Autodesk Inventor part; units mm, degrees
(part 5 of 8)
  spline S575 degree 2 poles (-11.5089, 13.7039) (-11.2834, 13.8253) (-11.2834, 14.1341) knots 0 0 0 1 1 1
  line L2030 (-11.5089, 13.7039) -> (-11.2834, 13.8253) construction
  line L2031 (-11.2834, 13.8253) -> (-11.2834, 14.1341) construction
  spline S576 degree 2 poles (-11.2834, 14.1341) (-11.2834, 14.4706) (-11.5297, 14.651) knots 0 0 0 1 1 1
  line L2032 (-11.2834, 14.1341) -> (-11.2834, 14.4706) construction
  line L2033 (-11.2834, 14.4706) -> (-11.5297, 14.651) construction
  line L2034 (-11.5297, 14.651) -> (-13.0701, 15.7924)
  spline S577 degree 2 poles (-13.0701, 15.7924) (-13.3546, 16.0006) (-13.3546, 16.3787) knots 0 0 0 1 1 1
  line L2035 (-13.0701, 15.7924) -> (-13.3546, 16.0006) construction
  line L2036 (-13.3546, 16.0006) -> (-13.3546, 16.3787) construction
  spline S578 degree 2 poles (-13.3546, 16.3787) (-13.3546, 16.8748) (-12.8932, 17.1177) knots 0 0 0 1 1 1
  line L2037 (-13.3546, 16.3787) -> (-13.3546, 16.8748) construction
  line L2038 (-13.3546, 16.8748) -> (-12.8932, 17.1177) construction
  spline S579 degree 2 poles (-12.8932, 17.1177) (-12.5601, 17.2877) (-12.1403, 17.2877) knots 0 0 0 1 1 1
  line L2039 (-12.8932, 17.1177) -> (-12.5601, 17.2877) construction
  line L2040 (-12.5601, 17.2877) -> (-12.1403, 17.2877) construction
  spline S580 degree 2 poles (-12.1403, 17.2877) (-11.5159, 17.2877) (-11.0232, 16.9373) knots 0 0 0 1 1 1
  line L2041 (-12.1403, 17.2877) -> (-11.5159, 17.2877) construction
  line L2042 (-11.5159, 17.2877) -> (-11.0232, 16.9373) construction
  spline S581 degree 2 poles (-11.0232, 16.9373) (-10.9295, 16.8714) (-10.9295, 16.7708) knots 0 0 0 1 1 1
  line L2043 (-11.0232, 16.9373) -> (-10.9295, 16.8714) construction
  line L2044 (-10.9295, 16.8714) -> (-10.9295, 16.7708) construction
  spline S582 degree 2 poles (-2.041, 23.007) (-1.9282, 23.007) (-1.7632, 23.172) (-1.7632, 23.2848) knots 0 0 0 1 2 2 2
  line L2045 (-2.041, 23.007) -> (-1.9282, 23.007) construction
  line L2046 (-1.9282, 23.007) -> (-1.7632, 23.172) construction
  line L2047 (-1.7632, 23.172) -> (-1.7632, 23.2848) construction
  line L2048 (-1.7632, 23.2848) -> (-1.7632, 24.2529)
  spline S583 degree 2 poles (-1.7632, 24.2529) (-1.7632, 24.3656) (-1.9282, 24.5306) (-2.041, 24.5306) knots 0 0 0 1 2 2 2
  line L2049 (-1.7632, 24.2529) -> (-1.7632, 24.3656) construction
  line L2050 (-1.7632, 24.3656) -> (-1.9282, 24.5306) construction
  line L2051 (-1.9282, 24.5306) -> (-2.041, 24.5306) construction
  spline S584 degree 2 poles (-2.6405, 21.8326) (-2.6405, 21.6236) (-2.8496, 21.6236) knots 0 0 0 1 1 1
  line L2052 (-2.6405, 21.8326) -> (-2.6405, 21.6236) construction
  line L2053 (-2.6405, 21.6236) -> (-2.8496, 21.6236) construction
  spline S585 degree 2 poles (-2.8496, 21.6236) (-3.0586, 21.6236) (-3.0586, 21.8326) knots 0 0 0 1 1 1
  line L2054 (-2.8496, 21.6236) -> (-3.0586, 21.6236) construction
  line L2055 (-3.0586, 21.6236) -> (-3.0586, 21.8326) construction
  line L2056 (-3.0586, 21.8326) -> (-3.0586, 24.7369)
  spline S586 degree 2 poles (-3.0586, 24.7369) (-3.0586, 24.9459) (-2.8496, 24.9459) knots 0 0 0 1 1 1
  line L2057 (-3.0586, 24.7369) -> (-3.0586, 24.9459) construction
  line L2058 (-3.0586, 24.9459) -> (-2.8496, 24.9459) construction
  line L2059 (-2.8496, 24.9459) -> (-2.041, 24.9459)
  spline S587 degree 2 poles (-2.041, 24.9459) (-1.7522, 24.9459) (-1.3452, 24.5389) (-1.3452, 24.2529) knots 0 0 0 1 2 2 2
  line L2060 (-2.041, 24.9459) -> (-1.7522, 24.9459) construction
  line L2061 (-1.7522, 24.9459) -> (-1.3452, 24.5389) construction
  line L2062 (-1.3452, 24.5389) -> (-1.3452, 24.2529) construction
  line L2063 (-1.3452, 24.2529) -> (-1.3452, 23.2848)
  spline S588 degree 2 poles (-1.3452, 23.2848) (-1.3452, 22.9987) (-1.7522, 22.5917) (-2.041, 22.5917) knots 0 0 0 1 2 2 2
  line L2064 (-1.3452, 23.2848) -> (-1.3452, 22.9987) construction
  line L2065 (-1.3452, 22.9987) -> (-1.7522, 22.5917) construction
  line L2066 (-1.7522, 22.5917) -> (-2.041, 22.5917) construction
  spline S589 degree 2 poles (0.2225, 23.007) (0.3353, 23.007) (0.5003, 23.172) (0.5003, 23.2848) knots 0 0 0 1 2 2 2
  line L2067 (0.2225, 23.007) -> (0.3353, 23.007) construction
  line L2068 (0.3353, 23.007) -> (0.5003, 23.172) construction
  line L2069 (0.5003, 23.172) -> (0.5003, 23.2848) construction
  spline S590 degree 2 poles (-0.102, 24.5306) (-0.2148, 24.5306) (-0.3771, 24.3684) (-0.3771, 24.2529) knots 0 0 0 1 2 2 2
  line L2070 (-0.102, 24.5306) -> (-0.2148, 24.5306) construction
  line L2071 (-0.2148, 24.5306) -> (-0.3771, 24.3684) construction
  line L2072 (-0.3771, 24.3684) -> (-0.3771, 24.2529) construction
  line L2073 (-0.3771, 24.2529) -> (-0.3771, 23.2848)
  spline S591 degree 2 poles (-0.3771, 23.2848) (-0.3771, 23.1693) (-0.2148, 23.007) (-0.102, 23.007) knots 0 0 0 1 2 2 2
  line L2074 (-0.3771, 23.2848) -> (-0.3771, 23.1693) construction
  line L2075 (-0.3771, 23.1693) -> (-0.2148, 23.007) construction
  line L2076 (-0.2148, 23.007) -> (-0.102, 23.007) construction
  line L2077 (-0.102, 23.007) -> (0.2225, 23.007)
  line L2078 (0.2225, 22.5917) -> (-0.102, 22.5917)
  spline S592 degree 2 poles (-0.102, 22.5917) (-0.3881, 22.5917) (-0.7951, 22.996) (-0.7951, 23.2848) knots 0 0 0 1 2 2 2
  line L2079 (-0.102, 22.5917) -> (-0.3881, 22.5917) construction
  line L2080 (-0.3881, 22.5917) -> (-0.7951, 22.996) construction
  line L2081 (-0.7951, 22.996) -> (-0.7951, 23.2848) construction
  line L2082 (-0.7951, 23.2848) -> (-0.7951, 24.2529)
  spline S593 degree 2 poles (-0.7951, 24.2529) (-0.7951, 24.5417) (-0.3853, 24.9459) (-0.102, 24.9459) knots 0 0 0 1 2 2 2
  line L2083 (-0.7951, 24.2529) -> (-0.7951, 24.5417) construction
  line L2084 (-0.7951, 24.5417) -> (-0.3853, 24.9459) construction
  line L2085 (-0.3853, 24.9459) -> (-0.102, 24.9459) construction
  line L2086 (-0.102, 24.9459) -> (0.7065, 24.9459)
  spline S594 degree 2 poles (0.7065, 24.9459) (0.9183, 24.9459) (0.9183, 24.7369) knots 0 0 0 1 1 1
  line L2087 (0.7065, 24.9459) -> (0.9183, 24.9459) construction
  line L2088 (0.9183, 24.9459) -> (0.9183, 24.7369) construction
  line L2089 (0.9183, 24.7369) -> (0.9183, 23.2875)
  spline S595 degree 2 poles (0.9183, 23.2875) (0.9183, 23.0758) (1.0751, 22.996) knots 0 0 0 1 1 1
  line L2090 (0.9183, 23.2875) -> (0.9183, 23.0758) construction
  line L2091 (0.9183, 23.0758) -> (1.0751, 22.996) construction
  spline S596 degree 2 poles (1.0751, 22.996) (1.2456, 22.9382) (1.2456, 22.8062) knots 0 0 0 1 1 1
  line L2092 (1.0751, 22.996) -> (1.2456, 22.9382) construction
  line L2093 (1.2456, 22.9382) -> (1.2456, 22.8062) construction
  spline S597 degree 2 poles (1.2456, 22.8062) (1.2456, 22.721) (1.1273, 22.589) (1.0366, 22.589) knots 0 0 0 1 2 2 2
  line L2094 (1.2456, 22.8062) -> (1.2456, 22.721) construction
  line L2095 (1.2456, 22.721) -> (1.1273, 22.589) construction
  line L2096 (1.1273, 22.589) -> (1.0366, 22.589) construction
  spline S598 degree 2 poles (1.0366, 22.589) (0.9898, 22.589) (0.9321, 22.6137) knots 0 0 0 1 1 1
  line L2097 (1.0366, 22.589) -> (0.9898, 22.589) construction
  line L2098 (0.9898, 22.589) -> (0.9321, 22.6137) construction
  spline S599 degree 2 poles (0.9321, 22.6137) (0.7725, 22.6852) (0.701, 22.8062) knots 0 0 0 1 1 1
  line L2099 (0.9321, 22.6137) -> (0.7725, 22.6852) construction
  line L2100 (0.7725, 22.6852) -> (0.701, 22.8062) construction
  spline S600 degree 2 poles (0.701, 22.8062) (0.5333, 22.5917) (0.2225, 22.5917) knots 0 0 0 1 1 1
  line L2101 (0.701, 22.8062) -> (0.5333, 22.5917) construction
  line L2102 (0.5333, 22.5917) -> (0.2225, 22.5917) construction
  spline S601 degree 2 poles (2.486, 23.007) (2.5987, 23.007) (2.7637, 23.172) (2.7637, 23.2848) knots 0 0 0 1 2 2 2
  line L2103 (2.486, 23.007) -> (2.5987, 23.007) construction
  line L2104 (2.5987, 23.007) -> (2.7637, 23.172) construction
  line L2105 (2.7637, 23.172) -> (2.7637, 23.2848) construction
  line L2106 (2.7637, 23.2848) -> (2.7637, 24.2529)
  spline S602 degree 2 poles (2.7637, 24.2529) (2.7637, 24.3656) (2.5987, 24.5306) (2.486, 24.5306) knots 0 0 0 1 2 2 2
  line L2107 (2.7637, 24.2529) -> (2.7637, 24.3656) construction
  line L2108 (2.7637, 24.3656) -> (2.5987, 24.5306) construction
  line L2109 (2.5987, 24.5306) -> (2.486, 24.5306) construction
  line L2110 (2.486, 24.5306) -> (2.1614, 24.5306)
  spline S603 degree 2 poles (2.1614, 24.5306) (2.0487, 24.5306) (1.8864, 24.3684) (1.8864, 24.2529) knots 0 0 0 1 2 2 2
  line L2111 (2.1614, 24.5306) -> (2.0487, 24.5306) construction
  line L2112 (2.0487, 24.5306) -> (1.8864, 24.3684) construction
  line L2113 (1.8864, 24.3684) -> (1.8864, 24.2529) construction
  line L2114 (1.8864, 24.2529) -> (1.8864, 23.2848)
  spline S604 degree 2 poles (1.8864, 23.2848) (1.8864, 23.1693) (2.0487, 23.007) (2.1614, 23.007) knots 0 0 0 1 2 2 2
  line L2115 (1.8864, 23.2848) -> (1.8864, 23.1693) construction
  line L2116 (1.8864, 23.1693) -> (2.0487, 23.007) construction
  line L2117 (2.0487, 23.007) -> (2.1614, 23.007) construction
  line L2118 (2.1614, 23.007) -> (2.486, 23.007)
  spline S605 degree 2 poles (1.5289, 25.5565) (1.4574, 25.628) (1.4574, 25.7215) knots 0 0 0 1 1 1
  line L2119 (1.5289, 25.5565) -> (1.4574, 25.628) construction
  line L2120 (1.4574, 25.628) -> (1.4574, 25.7215) construction
  spline S606 degree 2 poles (1.4574, 25.7215) (1.4574, 25.914) (1.6746, 25.914) knots 0 0 0 1 1 1
  line L2121 (1.4574, 25.7215) -> (1.4574, 25.914) construction
  line L2122 (1.4574, 25.914) -> (1.6746, 25.914) construction
  line L2123 (1.6746, 25.914) -> (2.97, 25.914)
  spline S607 degree 2 poles (2.97, 25.914) (3.1818, 25.914) (3.1818, 25.7078) knots 0 0 0 1 1 1
  line L2124 (2.97, 25.914) -> (3.1818, 25.914) construction
  line L2125 (3.1818, 25.914) -> (3.1818, 25.7078) construction
  spline S608 degree 2 poles (3.1818, 25.7078) (3.1818, 25.4987) (2.97, 25.4987) knots 0 0 0 1 1 1
  line L2126 (3.1818, 25.7078) -> (3.1818, 25.4987) construction
  line L2127 (3.1818, 25.4987) -> (2.97, 25.4987) construction
  spline S609 degree 2 poles (2.97, 24.7644) (3.0058, 24.7342) (3.0195, 24.6984) knots 0 0 0 1 1 1
  line L2128 (2.97, 24.7644) -> (3.0058, 24.7342) construction
  line L2129 (3.0058, 24.7342) -> (3.0195, 24.6984) construction
  spline S610 degree 2 poles (3.0195, 24.6984) (3.1818, 24.5114) (3.1818, 24.2529) knots 0 0 0 1 1 1
  line L2130 (3.0195, 24.6984) -> (3.1818, 24.5114) construction
  line L2131 (3.1818, 24.5114) -> (3.1818, 24.2529) construction
  line L2132 (3.1818, 24.2529) -> (3.1818, 23.2848)
  spline S611 degree 2 poles (3.1818, 23.2848) (3.1818, 22.9987) (2.7747, 22.5917) (2.486, 22.5917) knots 0 0 0 1 2 2 2
  line L2133 (3.1818, 23.2848) -> (3.1818, 22.9987) construction
  line L2134 (3.1818, 22.9987) -> (2.7747, 22.5917) construction
  line L2135 (2.7747, 22.5917) -> (2.486, 22.5917) construction
  line L2136 (2.486, 22.5917) -> (2.1614, 22.5917)
  spline S612 degree 2 poles (2.1614, 22.5917) (1.8754, 22.5917) (1.4684, 22.996) (1.4684, 23.2848) knots 0 0 0 1 2 2 2
  line L2137 (2.1614, 22.5917) -> (1.8754, 22.5917) construction
  line L2138 (1.8754, 22.5917) -> (1.4684, 22.996) construction
  line L2139 (1.4684, 22.996) -> (1.4684, 23.2848) construction
  line L2140 (1.4684, 23.2848) -> (1.4684, 24.2529)
  spline S613 degree 2 poles (1.4684, 24.2529) (1.4684, 24.5417) (1.8782, 24.9459) (2.1614, 24.9459) knots 0 0 0 1 2 2 2
  line L2141 (1.4684, 24.2529) -> (1.4684, 24.5417) construction
  line L2142 (1.4684, 24.5417) -> (1.8782, 24.9459) construction
  line L2143 (1.8782, 24.9459) -> (2.1614, 24.9459) construction
  spline S614 degree 2 poles (10.5768, 22.5747) (10.2935, 22.5747) (9.8864, 22.979) (9.8864, 23.2678) knots 0 0 0 1 2 2 2
  line L2144 (10.5768, 22.5747) -> (10.2935, 22.5747) construction
  line L2145 (10.2935, 22.5747) -> (9.8864, 22.979) construction
  line L2146 (9.8864, 22.979) -> (9.8864, 23.2678) construction
  line L2147 (9.8864, 23.2678) -> (9.8864, 24.2359)
  spline S615 degree 2 poles (9.8864, 24.2359) (9.8864, 24.5246) (10.2935, 24.9289) (10.5768, 24.9289) knots 0 0 0 1 2 2 2
  line L2148 (9.8864, 24.2359) -> (9.8864, 24.5246) construction
  line L2149 (9.8864, 24.5246) -> (10.2935, 24.9289) construction
  line L2150 (10.2935, 24.9289) -> (10.5768, 24.9289) construction
  line L2151 (10.5768, 24.9289) -> (11.0608, 24.9289)
  spline S616 degree 2 poles (11.0608, 24.9289) (11.2726, 24.9289) (11.2726, 24.7227) knots 0 0 0 1 1 1
  line L2152 (11.0608, 24.9289) -> (11.2726, 24.9289) construction
  line L2153 (11.2726, 24.9289) -> (11.2726, 24.7227) construction
  spline S617 degree 2 poles (11.2726, 24.7227) (11.2726, 24.5136) (11.0608, 24.5136) knots 0 0 0 1 1 1
  line L2154 (11.2726, 24.7227) -> (11.2726, 24.5136) construction
  line L2155 (11.2726, 24.5136) -> (11.0608, 24.5136) construction
  line L2156 (11.0608, 24.5136) -> (10.5768, 24.5136)
  spline S618 degree 2 poles (10.5768, 24.5136) (10.4667, 24.5136) (10.3045, 24.3514) (10.3045, 24.2359) knots 0 0 0 1 2 2 2
  line L2157 (10.5768, 24.5136) -> (10.4667, 24.5136) construction
  line L2158 (10.4667, 24.5136) -> (10.3045, 24.3514) construction
  line L2159 (10.3045, 24.3514) -> (10.3045, 24.2359) construction
  line L2160 (10.3045, 24.2359) -> (10.3045, 23.2678)
  spline S619 degree 2 poles (10.3045, 23.2678) (10.3045, 23.1523) (10.4667, 22.99) (10.5768, 22.99) knots 0 0 0 1 2 2 2
  line L2161 (10.3045, 23.2678) -> (10.3045, 23.1523) construction
  line L2162 (10.3045, 23.1523) -> (10.4667, 22.99) construction
  line L2163 (10.4667, 22.99) -> (10.5768, 22.99) construction
  line L2164 (10.5768, 22.99) -> (11.0608, 22.99)
  spline S620 degree 2 poles (11.0608, 22.99) (11.2726, 22.99) (11.2726, 22.7837) knots 0 0 0 1 1 1
  line L2165 (11.0608, 22.99) -> (11.2726, 22.99) construction
  line L2166 (11.2726, 22.99) -> (11.2726, 22.7837) construction
  spline S621 degree 2 poles (11.2726, 22.7837) (11.2726, 22.5747) (11.0608, 22.5747) knots 0 0 0 1 1 1
  line L2167 (11.2726, 22.7837) -> (11.2726, 22.5747) construction
  line L2168 (11.2726, 22.5747) -> (11.0608, 22.5747) construction
  line L2169 (11.0608, 22.5747) -> (10.5768, 22.5747)
  spline S622 degree 2 poles (14.7819, 22.5747) (14.4959, 22.5747) (14.0861, 22.979) (14.0861, 23.2678) knots 0 0 0 1 2 2 2
  line L2170 (14.7819, 22.5747) -> (14.4959, 22.5747) construction
  line L2171 (14.4959, 22.5747) -> (14.0861, 22.979) construction
  line L2172 (14.0861, 22.979) -> (14.0861, 23.2678) construction
  line L2173 (14.0861, 23.2678) -> (14.0861, 24.7199)
  spline S623 degree 2 poles (14.0861, 24.7199) (14.0861, 24.9289) (14.2951, 24.9289) knots 0 0 0 1 1 1
  line L2174 (14.0861, 24.7199) -> (14.0861, 24.9289) construction
  line L2175 (14.0861, 24.9289) -> (14.2951, 24.9289) construction
  spline S624 degree 2 poles (14.2951, 24.9289) (14.5041, 24.9289) (14.5041, 24.7199) knots 0 0 0 1 1 1
  line L2176 (14.2951, 24.9289) -> (14.5041, 24.9289) construction
  line L2177 (14.5041, 24.9289) -> (14.5041, 24.7199) construction
  line L2178 (14.5041, 24.7199) -> (14.5041, 23.2678)
  spline S625 degree 2 poles (14.5041, 23.2678) (14.5041, 23.1523) (14.6664, 22.99) (14.7792, 22.99) knots 0 0 0 1 2 2 2
  line L2179 (14.5041, 23.2678) -> (14.5041, 23.1523) construction
  line L2180 (14.5041, 23.1523) -> (14.6664, 22.99) construction
  line L2181 (14.6664, 22.99) -> (14.7792, 22.99) construction
  spline S626 degree 2 poles (15.3815, 24.7199) (15.3815, 24.9289) (15.5905, 24.9289) knots 0 0 0 1 1 1
  line L2182 (15.3815, 24.7199) -> (15.3815, 24.9289) construction
  line L2183 (15.3815, 24.9289) -> (15.5905, 24.9289) construction
  spline S627 degree 2 poles (15.5905, 24.9289) (15.7995, 24.9289) (15.7995, 24.7199) knots 0 0 0 1 1 1
  line L2184 (15.5905, 24.9289) -> (15.7995, 24.9289) construction
  line L2185 (15.7995, 24.9289) -> (15.7995, 24.7199) construction
  line L2186 (15.7995, 24.7199) -> (15.7995, 22.2997)
  spline S628 degree 2 poles (15.7995, 22.2997) (15.7995, 22.0109) (15.3925, 21.6066) (15.1037, 21.6066) knots 0 0 0 1 2 2 2
  line L2187 (15.7995, 22.2997) -> (15.7995, 22.0109) construction
  line L2188 (15.7995, 22.0109) -> (15.3925, 21.6066) construction
  line L2189 (15.3925, 21.6066) -> (15.1037, 21.6066) construction
  line L2190 (15.1037, 21.6066) -> (14.4546, 21.6066)
  spline S629 degree 2 poles (14.4546, 21.6066) (14.2456, 21.6066) (14.2456, 21.8156) knots 0 0 0 1 1 1
  line L2191 (14.4546, 21.6066) -> (14.2456, 21.6066) construction
  line L2192 (14.2456, 21.6066) -> (14.2456, 21.8156) construction
  spline S630 degree 2 poles (14.2456, 21.8156) (14.2456, 22.0219) (14.4546, 22.0219) knots 0 0 0 1 1 1
  line L2193 (14.2456, 21.8156) -> (14.2456, 22.0219) construction
  line L2194 (14.2456, 22.0219) -> (14.4546, 22.0219) construction
  line L2195 (14.4546, 22.0219) -> (15.1037, 22.0219)
  spline S631 degree 2 poles (15.1037, 22.0219) (15.2165, 22.0219) (15.3815, 22.1869) (15.3815, 22.2997) knots 0 0 0 1 2 2 2
  line L2196 (15.1037, 22.0219) -> (15.2165, 22.0219) construction
  line L2197 (15.2165, 22.0219) -> (15.3815, 22.1869) construction
  line L2198 (15.3815, 22.1869) -> (15.3815, 22.2997) construction
  spline S632 degree 2 poles (19.4656, 22.99) (19.6747, 22.99) (19.6747, 22.7837) knots 0 0 0 1 1 1
  line L2199 (19.4656, 22.99) -> (19.6747, 22.99) construction
  line L2200 (19.6747, 22.99) -> (19.6747, 22.7837) construction
  spline S633 degree 2 poles (19.6747, 22.7837) (19.6747, 22.5747) (19.4656, 22.5747) knots 0 0 0 1 1 1
  line L2201 (19.6747, 22.7837) -> (19.6747, 22.5747) construction
  line L2202 (19.6747, 22.5747) -> (19.4656, 22.5747) construction
  spline S634 degree 2 poles (19.4656, 22.5747) (19.2566, 22.5747) (19.2566, 22.7837) knots 0 0 0 1 1 1
  line L2203 (19.4656, 22.5747) -> (19.2566, 22.5747) construction
  line L2204 (19.2566, 22.5747) -> (19.2566, 22.7837) construction
  spline S635 degree 2 poles (19.2566, 22.7837) (19.2566, 22.99) (19.4656, 22.99) knots 0 0 0 1 1 1
  line L2205 (19.2566, 22.7837) -> (19.2566, 22.99) construction
  line L2206 (19.2566, 22.99) -> (19.4656, 22.99) construction
  spline S636 degree 2 poles (-14.6719, -1.3741) (-14.5019, -1.3741) (-14.2591, -1.1278) (-14.2591, -0.9578) knots 0 0 0 1 2 2 2
  line L2207 (-14.6719, -1.3741) -> (-14.5019, -1.3741) construction
  line L2208 (-14.5019, -1.3741) -> (-14.2591, -1.1278) construction
  line L2209 (-14.2591, -1.1278) -> (-14.2591, -0.9578) construction
  spline S637 degree 2 poles (-15.0883, 0.7006) (-15.2582, 0.7006) (-15.5011, 0.4542) (-15.5011, 0.2842) knots 0 0 0 1 2 2 2
  line L2210 (-15.0883, 0.7006) -> (-15.2582, 0.7006) construction
  line L2211 (-15.2582, 0.7006) -> (-15.5011, 0.4542) construction
  line L2212 (-15.5011, 0.4542) -> (-15.5011, 0.2842) construction
  line L2213 (-15.5011, 0.2842) -> (-15.5011, -0.9578)
  spline S638 degree 2 poles (-15.5011, -0.9578) (-15.5011, -1.1278) (-15.2582, -1.3741) (-15.0883, -1.3741) knots 0 0 0 1 2 2 2
  line L2214 (-15.5011, -0.9578) -> (-15.5011, -1.1278) construction
  line L2215 (-15.5011, -1.1278) -> (-15.2582, -1.3741) construction
  line L2216 (-15.2582, -1.3741) -> (-15.0883, -1.3741) construction
  line L2217 (-15.0883, -1.3741) -> (-14.6719, -1.3741)
  line L2218 (-14.6719, -1.7904) -> (-15.0883, -1.7904)
  spline S639 degree 2 poles (-15.0883, -1.7904) (-15.4282, -1.7904) (-15.9174, -1.3047) (-15.9174, -0.9612) knots 0 0 0 1 2 2 2
  line L2219 (-15.0883, -1.7904) -> (-15.4282, -1.7904) construction
  line L2220 (-15.4282, -1.7904) -> (-15.9174, -1.3047) construction
  line L2221 (-15.9174, -1.3047) -> (-15.9174, -0.9612) construction
  line L2222 (-15.9174, -0.9612) -> (-15.9174, 0.2877)
  spline S640 degree 2 poles (-15.9174, 0.2877) (-15.9174, 0.6312) (-15.4282, 1.1169) (-15.0883, 1.1169) knots 0 0 0 1 2 2 2
  line L2223 (-15.9174, 0.2877) -> (-15.9174, 0.6312) construction
  line L2224 (-15.9174, 0.6312) -> (-15.4282, 1.1169) construction
  line L2225 (-15.4282, 1.1169) -> (-15.0883, 1.1169) construction
  line L2226 (-15.0883, 1.1169) -> (-14.0509, 1.1169)
  spline S641 degree 2 poles (-14.0509, 1.1169) (-13.8428, 1.1169) (-13.8428, 0.9087) knots 0 0 0 1 1 1
  line L2227 (-14.0509, 1.1169) -> (-13.8428, 1.1169) construction
  line L2228 (-13.8428, 1.1169) -> (-13.8428, 0.9087) construction
  line L2229 (-13.8428, 0.9087) -> (-13.8428, -0.9543)
  spline S642 degree 2 poles (-13.8428, -0.9543) (-13.8428, -1.2665) (-13.5513, -1.3914) knots 0 0 0 1 1 1
  line L2230 (-13.8428, -0.9543) -> (-13.8428, -1.2665) construction
  line L2231 (-13.8428, -1.2665) -> (-13.5513, -1.3914) construction
  spline S643 degree 2 poles (-13.5513, -1.3914) (-13.423, -1.4435) (-13.423, -1.5753) knots 0 0 0 1 1 1
  line L2232 (-13.5513, -1.3914) -> (-13.423, -1.4435) construction
  line L2233 (-13.423, -1.4435) -> (-13.423, -1.5753) construction
  spline S644 degree 2 poles (-13.423, -1.5753) (-13.423, -1.662) (-13.5409, -1.7939) (-13.6277, -1.7939) knots 0 0 0 1 2 2 2
  line L2234 (-13.423, -1.5753) -> (-13.423, -1.662) construction
  line L2235 (-13.423, -1.662) -> (-13.5409, -1.7939) construction
  line L2236 (-13.5409, -1.7939) -> (-13.6277, -1.7939) construction
  spline S645 degree 2 poles (-13.6277, -1.7939) (-13.6728, -1.7939) (-13.7179, -1.7731) knots 0 0 0 1 1 1
  line L2237 (-13.6277, -1.7939) -> (-13.6728, -1.7939) construction
  line L2238 (-13.6728, -1.7939) -> (-13.7179, -1.7731) construction
  spline S646 degree 2 poles (-13.7179, -1.7731) (-13.926, -1.6829) (-14.0544, -1.5163) knots 0 0 0 1 1 1
  line L2239 (-13.7179, -1.7731) -> (-13.926, -1.6829) construction
  line L2240 (-13.926, -1.6829) -> (-14.0544, -1.5163) construction
  spline S647 degree 2 poles (-14.0544, -1.5163) (-14.3042, -1.7904) (-14.6719, -1.7904) knots 0 0 0 1 1 1
  line L2241 (-14.0544, -1.5163) -> (-14.3042, -1.7904) construction
  line L2242 (-14.3042, -1.7904) -> (-14.6719, -1.7904) construction
  spline S648 degree 2 poles (-11.1436, -1.7904) (-11.3518, -1.7904) (-11.3518, -1.5823) knots 0 0 0 1 1 1
  line L2243 (-11.1436, -1.7904) -> (-11.3518, -1.7904) construction
  line L2244 (-11.3518, -1.7904) -> (-11.3518, -1.5823) construction
  line L2245 (-11.3518, -1.5823) -> (-11.3518, 0.2842)
  spline S649 degree 2 poles (-11.3518, 0.2842) (-11.3518, 0.4542) (-11.5946, 0.7006) (-11.7646, 0.7006) knots 0 0 0 1 2 2 2
  line L2246 (-11.3518, 0.2842) -> (-11.3518, 0.4542) construction
  line L2247 (-11.3518, 0.4542) -> (-11.5946, 0.7006) construction
  line L2248 (-11.5946, 0.7006) -> (-11.7646, 0.7006) construction
  spline S650 degree 2 poles (-12.5938, -1.5823) (-12.5938, -1.7904) (-12.802, -1.7904) knots 0 0 0 1 1 1
  line L2249 (-12.5938, -1.5823) -> (-12.5938, -1.7904) construction
  line L2250 (-12.5938, -1.7904) -> (-12.802, -1.7904) construction
  spline S651 degree 2 poles (-12.802, -1.7904) (-13.0101, -1.7904) (-13.0101, -1.5823) knots 0 0 0 1 1 1
  line L2251 (-12.802, -1.7904) -> (-13.0101, -1.7904) construction
  line L2252 (-13.0101, -1.7904) -> (-13.0101, -1.5823) construction
  line L2253 (-13.0101, -1.5823) -> (-13.0101, 0.9087)
  spline S652 degree 2 poles (-13.0101, 0.9087) (-13.0101, 1.1169) (-12.802, 1.1169) knots 0 0 0 1 1 1
  line L2254 (-13.0101, 0.9087) -> (-13.0101, 1.1169) construction
  line L2255 (-13.0101, 1.1169) -> (-12.802, 1.1169) construction
  line L2256 (-12.802, 1.1169) -> (-11.7646, 1.1169)
  spline S653 degree 2 poles (-11.7646, 1.1169) (-11.4212, 1.1169) (-10.9355, 0.6312) (-10.9355, 0.2877) knots 0 0 0 1 2 2 2
  line L2257 (-11.7646, 1.1169) -> (-11.4212, 1.1169) construction
  line L2258 (-11.4212, 1.1169) -> (-10.9355, 0.6312) construction
  line L2259 (-10.9355, 0.6312) -> (-10.9355, 0.2877) construction
  line L2260 (-10.9355, 0.2877) -> (-10.9355, -1.5823)
  spline S654 degree 2 poles (-10.9355, -1.5823) (-10.9355, -1.7904) (-11.1436, -1.7904) knots 0 0 0 1 1 1
  line L2261 (-10.9355, -1.5823) -> (-10.9355, -1.7904) construction
  line L2262 (-10.9355, -1.7904) -> (-11.1436, -1.7904) construction
  spline S655 degree 2 poles (-13.0931, 3.6508) (-13.2111, 3.6508) (-13.2735, 3.7618) knots 0 0 0 1 1 1
  line L2263 (-13.0931, 3.6508) -> (-13.2111, 3.6508) construction
  line L2264 (-13.2111, 3.6508) -> (-13.2735, 3.7618) construction
  spline S656 degree 2 poles (-14.9839, 3.8624) (-14.9839, 3.6542) (-15.1921, 3.6542) knots 0 0 0 1 1 1
  line L2265 (-14.9839, 3.8624) -> (-14.9839, 3.6542) construction
  line L2266 (-14.9839, 3.6542) -> (-15.1921, 3.6542) construction
  spline S657 degree 2 poles (-15.1921, 3.6542) (-15.4002, 3.6542) (-15.4002, 3.8624) knots 0 0 0 1 1 1
  line L2267 (-15.1921, 3.6542) -> (-15.4002, 3.6542) construction
  line L2268 (-15.4002, 3.6542) -> (-15.4002, 3.8624) construction
  line L2269 (-15.4002, 3.8624) -> (-15.4002, 7.5989)
  spline S658 degree 2 poles (-15.4002, 7.5989) (-15.4002, 7.8035) (-15.1921, 7.8035) knots 0 0 0 1 1 1
  line L2270 (-15.4002, 7.5989) -> (-15.4002, 7.8035) construction
  line L2271 (-15.4002, 7.8035) -> (-15.1921, 7.8035) construction
  spline S659 degree 2 poles (-15.1921, 7.8035) (-14.9839, 7.8035) (-14.9839, 7.5989) knots 0 0 0 1 1 1
  line L2272 (-15.1921, 7.8035) -> (-14.9839, 7.8035) construction
  line L2273 (-14.9839, 7.8035) -> (-14.9839, 7.5989) construction
  spline S660 degree 2 poles (-13.2354, 7.7446) (-13.1729, 7.807) (-13.0931, 7.807) knots 0 0 0 1 1 1
  line L2274 (-13.2354, 7.7446) -> (-13.1729, 7.807) construction
  line L2275 (-13.1729, 7.807) -> (-13.0931, 7.807) construction
  spline S661 degree 2 poles (-13.0931, 7.807) (-13.0099, 7.807) (-12.8815, 7.6787) (-12.8815, 7.5954) knots 0 0 0 1 2 2 2
  line L2276 (-13.0931, 7.807) -> (-13.0099, 7.807) construction
  line L2277 (-13.0099, 7.807) -> (-12.8815, 7.6787) construction
  line L2278 (-12.8815, 7.6787) -> (-12.8815, 7.5954) construction
  spline S662 degree 2 poles (-12.8815, 7.5954) (-12.8815, 7.5156) (-12.9439, 7.4531) knots 0 0 0 1 1 1
  line L2279 (-12.8815, 7.5954) -> (-12.8815, 7.5156) construction
  line L2280 (-12.8815, 7.5156) -> (-12.9439, 7.4531) construction
  spline S663 degree 2 poles (-12.9058, 3.963) (-12.878, 3.9075) (-12.878, 3.8554) knots 0 0 0 1 1 1
  line L2281 (-12.9058, 3.963) -> (-12.878, 3.9075) construction
  line L2282 (-12.878, 3.9075) -> (-12.878, 3.8554) construction
  spline S664 degree 2 poles (-12.878, 3.8554) (-12.878, 3.7722) (-13.0099, 3.6508) (-13.0931, 3.6508) knots 0 0 0 1 2 2 2
  line L2283 (-12.878, 3.8554) -> (-12.878, 3.7722) construction
  line L2284 (-12.878, 3.7722) -> (-13.0099, 3.6508) construction
  line L2285 (-13.0099, 3.6508) -> (-13.0931, 3.6508) construction
  spline S665 degree 2 poles (-15.0713, -10.8765) (-15.505, -10.8765) (-16.1121, -10.2694) (-16.1121, -9.8392) knots 0 0 0 1 2 2 2
  line L2286 (-15.0713, -10.8765) -> (-15.505, -10.8765) construction
  line L2287 (-15.505, -10.8765) -> (-16.1121, -10.2694) construction
  line L2288 (-16.1121, -10.2694) -> (-16.1121, -9.8392) construction
  line L2289 (-16.1121, -9.8392) -> (-16.1121, -7.7611)
  spline S666 degree 2 poles (-16.1121, -7.7611) (-16.1121, -7.3343) (-15.505, -6.7237) (-15.0713, -6.7237) knots 0 0 0 1 2 2 2
  line L2290 (-16.1121, -7.7611) -> (-16.1121, -7.3343) construction
  line L2291 (-16.1121, -7.3343) -> (-15.505, -6.7237) construction
  line L2292 (-15.505, -6.7237) -> (-15.0713, -6.7237) construction
  line L2293 (-15.0713, -6.7237) -> (-14.2421, -6.7237)
  spline S667 degree 2 poles (-14.2421, -6.7237) (-14.034, -6.7237) (-14.034, -6.9319) knots 0 0 0 1 1 1
  line L2294 (-14.2421, -6.7237) -> (-14.034, -6.7237) construction
  line L2295 (-14.034, -6.7237) -> (-14.034, -6.9319) construction
  spline S668 degree 2 poles (-14.034, -6.9319) (-14.034, -7.1401) (-14.2421, -7.1401) knots 0 0 0 1 1 1
  line L2296 (-14.034, -6.9319) -> (-14.034, -7.1401) construction
  line L2297 (-14.034, -7.1401) -> (-14.2421, -7.1401) construction
  line L2298 (-14.2421, -7.1401) -> (-15.0713, -7.1401)
  spline S669 degree 2 poles (-15.0713, -7.1401) (-15.3315, -7.1401) (-15.6958, -7.5043) (-15.6958, -7.7611) knots 0 0 0 1 2 2 2
  line L2299 (-15.0713, -7.1401) -> (-15.3315, -7.1401) construction
  line L2300 (-15.3315, -7.1401) -> (-15.6958, -7.5043) construction
  line L2301 (-15.6958, -7.5043) -> (-15.6958, -7.7611) construction
  line L2302 (-15.6958, -7.7611) -> (-15.6958, -9.8392)
  spline S670 degree 2 poles (-15.6958, -9.8392) (-15.6958, -10.0959) (-15.3315, -10.4602) (-15.0713, -10.4602) knots 0 0 0 1 2 2 2
  line L2303 (-15.6958, -9.8392) -> (-15.6958, -10.0959) construction
  line L2304 (-15.6958, -10.0959) -> (-15.3315, -10.4602) construction
  line L2305 (-15.3315, -10.4602) -> (-15.0713, -10.4602) construction
  line L2306 (-15.0713, -10.4602) -> (-14.2421, -10.4602)
  spline S671 degree 2 poles (-14.2421, -10.4602) (-14.034, -10.4602) (-14.034, -10.6684) knots 0 0 0 1 1 1
  line L2307 (-14.2421, -10.4602) -> (-14.034, -10.4602) construction
  line L2308 (-14.034, -10.4602) -> (-14.034, -10.6684) construction
  spline S672 degree 2 poles (-14.034, -10.6684) (-14.034, -10.8765) (-14.2421, -10.8765) knots 0 0 0 1 1 1
  line L2309 (-14.034, -10.6684) -> (-14.034, -10.8765) construction
  line L2310 (-14.034, -10.8765) -> (-14.2421, -10.8765) construction
  line L2311 (-14.2421, -10.8765) -> (-15.0713, -10.8765)
  spline S673 degree 2 poles (-7.5984, -10.8765) (-7.8065, -10.8765) (-7.8065, -10.6684) knots 0 0 0 1 1 1
  line L2312 (-7.5984, -10.8765) -> (-7.8065, -10.8765) construction
  line L2313 (-7.8065, -10.8765) -> (-7.8065, -10.6684) construction
  spline S674 degree 2 poles (-9.4649, -10.6684) (-9.4649, -10.8765) (-9.673, -10.8765) knots 0 0 0 1 1 1
  line L2314 (-9.4649, -10.6684) -> (-9.4649, -10.8765) construction
  line L2315 (-9.4649, -10.8765) -> (-9.673, -10.8765) construction
  spline S675 degree 2 poles (-9.673, -10.8765) (-9.8812, -10.8765) (-9.8812, -10.6684) knots 0 0 0 1 1 1
  line L2316 (-9.673, -10.8765) -> (-9.8812, -10.8765) construction
  line L2317 (-9.8812, -10.8765) -> (-9.8812, -10.6684) construction
  line L2318 (-9.8812, -10.6684) -> (-9.8812, -6.9319)
  spline S676 degree 2 poles (-9.8812, -6.9319) (-9.8812, -6.7237) (-9.673, -6.7237) knots 0 0 0 1 1 1
  line L2319 (-9.8812, -6.9319) -> (-9.8812, -6.7237) construction
  line L2320 (-9.8812, -6.7237) -> (-9.673, -6.7237) construction
  line L2321 (-9.673, -6.7237) -> (-7.5984, -6.7237)
  spline S677 degree 2 poles (-7.5984, -6.7237) (-7.3902, -6.7237) (-7.3902, -6.9319) knots 0 0 0 1 1 1
  line L2322 (-7.5984, -6.7237) -> (-7.3902, -6.7237) construction
  line L2323 (-7.3902, -6.7237) -> (-7.3902, -6.9319) construction
  line L2324 (-7.3902, -6.9319) -> (-7.3902, -10.6684)
  spline S678 degree 2 poles (-7.3902, -10.6684) (-7.3902, -10.8765) (-7.5984, -10.8765) knots 0 0 0 1 1 1
  line L2325 (-7.3902, -10.6684) -> (-7.3902, -10.8765) construction
  line L2326 (-7.3902, -10.8765) -> (-7.5984, -10.8765) construction
  spline S679 degree 2 poles (9.7601, -1.2577) (9.9301, -1.2577) (10.1729, -1.0114) (10.1729, -0.8414) knots 0 0 0 1 2 2 2
  line L2327 (9.7601, -1.2577) -> (9.9301, -1.2577) construction
  line L2328 (9.9301, -1.2577) -> (10.1729, -1.0114) construction
  line L2329 (10.1729, -1.0114) -> (10.1729, -0.8414) construction
  spline S680 degree 2 poles (9.3438, 0.8169) (9.1738, 0.8169) (8.9309, 0.5706) (8.9309, 0.4006) knots 0 0 0 1 2 2 2
  line L2330 (9.3438, 0.8169) -> (9.1738, 0.8169) construction
  line L2331 (9.1738, 0.8169) -> (8.9309, 0.5706) construction
  line L2332 (8.9309, 0.5706) -> (8.9309, 0.4006) construction
  line L2333 (8.9309, 0.4006) -> (8.9309, -0.8414)
  spline S681 degree 2 poles (8.9309, -0.8414) (8.9309, -1.0114) (9.1738, -1.2577) (9.3438, -1.2577) knots 0 0 0 1 2 2 2
  line L2334 (8.9309, -0.8414) -> (8.9309, -1.0114) construction
  line L2335 (8.9309, -1.0114) -> (9.1738, -1.2577) construction
  line L2336 (9.1738, -1.2577) -> (9.3438, -1.2577) construction
  line L2337 (9.3438, -1.2577) -> (9.7601, -1.2577)
  line L2338 (9.7601, -1.674) -> (9.3438, -1.674)
  spline S682 degree 2 poles (9.3438, -1.674) (9.0038, -1.674) (8.5146, -1.1883) (8.5146, -0.8449) knots 0 0 0 1 2 2 2
  line L2339 (9.3438, -1.674) -> (9.0038, -1.674) construction
  line L2340 (9.0038, -1.674) -> (8.5146, -1.1883) construction
  line L2341 (8.5146, -1.1883) -> (8.5146, -0.8449) construction
  line L2342 (8.5146, -0.8449) -> (8.5146, 0.4041)
  spline S683 degree 2 poles (8.5146, 0.4041) (8.5146, 0.7475) (9.0038, 1.2333) (9.3438, 1.2333) knots 0 0 0 1 2 2 2
  line L2343 (8.5146, 0.4041) -> (8.5146, 0.7475) construction
  line L2344 (8.5146, 0.7475) -> (9.0038, 1.2333) construction
  line L2345 (9.0038, 1.2333) -> (9.3438, 1.2333) construction
  line L2346 (9.3438, 1.2333) -> (10.3811, 1.2333)
  spline S684 degree 2 poles (10.3811, 1.2333) (10.5893, 1.2333) (10.5893, 1.0251) knots 0 0 0 1 1 1
  line L2347 (10.3811, 1.2333) -> (10.5893, 1.2333) construction
  line L2348 (10.5893, 1.2333) -> (10.5893, 1.0251) construction
  line L2349 (10.5893, 1.0251) -> (10.5893, -0.8379)
  spline S685 degree 2 poles (10.5893, -0.8379) (10.5893, -1.1502) (10.8807, -1.2751) knots 0 0 0 1 1 1
  line L2350 (10.5893, -0.8379) -> (10.5893, -1.1502) construction
  line L2351 (10.5893, -1.1502) -> (10.8807, -1.2751) construction
  spline S686 degree 2 poles (10.8807, -1.2751) (11.009, -1.3271) (11.009, -1.4589) knots 0 0 0 1 1 1
  line L2352 (10.8807, -1.2751) -> (11.009, -1.3271) construction
  line L2353 (11.009, -1.3271) -> (11.009, -1.4589) construction
  spline S687 degree 2 poles (11.009, -1.4589) (11.009, -1.5457) (10.8911, -1.6775) (10.8044, -1.6775) knots 0 0 0 1 2 2 2
  line L2354 (11.009, -1.4589) -> (11.009, -1.5457) construction
  line L2355 (11.009, -1.5457) -> (10.8911, -1.6775) construction
  line L2356 (10.8911, -1.6775) -> (10.8044, -1.6775) construction
  spline S688 degree 2 poles (10.8044, -1.6775) (10.7593, -1.6775) (10.7142, -1.6567) knots 0 0 0 1 1 1
  line L2357 (10.8044, -1.6775) -> (10.7593, -1.6775) construction
  line L2358 (10.7593, -1.6775) -> (10.7142, -1.6567) construction
  spline S689 degree 2 poles (10.7142, -1.6567) (10.506, -1.5665) (10.3776, -1.4) knots 0 0 0 1 1 1
  line L2359 (10.7142, -1.6567) -> (10.506, -1.5665) construction
  line L2360 (10.506, -1.5665) -> (10.3776, -1.4) construction
  spline S690 degree 2 poles (10.3776, -1.4) (10.1278, -1.674) (9.7601, -1.674) knots 0 0 0 1 1 1
  line L2361 (10.3776, -1.4) -> (10.1278, -1.674) construction
  line L2362 (10.1278, -1.674) -> (9.7601, -1.674) construction
  spline S691 degree 2 poles (12.6674, -1.2577) (12.8374, -1.2577) (13.0802, -1.0114) (13.0802, -0.8414) knots 0 0 0 1 2 2 2
  line L2363 (12.6674, -1.2577) -> (12.8374, -1.2577) construction
  line L2364 (12.8374, -1.2577) -> (13.0802, -1.0114) construction
  line L2365 (13.0802, -1.0114) -> (13.0802, -0.8414) construction
  line L2366 (13.0802, -0.8414) -> (13.0802, 0.4006)
  spline S692 degree 2 poles (13.0802, 0.4006) (13.0802, 0.5706) (12.8374, 0.8169) (12.6674, 0.8169) knots 0 0 0 1 2 2 2
  line L2367 (13.0802, 0.4006) -> (13.0802, 0.5706) construction
  line L2368 (13.0802, 0.5706) -> (12.8374, 0.8169) construction
  line L2369 (12.8374, 0.8169) -> (12.6674, 0.8169) construction
  spline S693 degree 2 poles (11.8382, -2.7114) (11.8382, -2.9195) (11.6301, -2.9195) knots 0 0 0 1 1 1
  line L2370 (11.8382, -2.7114) -> (11.8382, -2.9195) construction
  line L2371 (11.8382, -2.9195) -> (11.6301, -2.9195) construction
  spline S694 degree 2 poles (11.6301, -2.9195) (11.4219, -2.9195) (11.4219, -2.7114) knots 0 0 0 1 1 1
  line L2372 (11.6301, -2.9195) -> (11.4219, -2.9195) construction
  line L2373 (11.4219, -2.9195) -> (11.4219, -2.7114) construction
  line L2374 (11.4219, -2.7114) -> (11.4219, 1.0251)
  spline S695 degree 2 poles (11.4219, 1.0251) (11.4219, 1.2333) (11.6301, 1.2333) knots 0 0 0 1 1 1
  line L2375 (11.4219, 1.0251) -> (11.4219, 1.2333) construction
  line L2376 (11.4219, 1.2333) -> (11.6301, 1.2333) construction
  line L2377 (11.6301, 1.2333) -> (12.6674, 1.2333)
  spline S696 degree 2 poles (12.6674, 1.2333) (13.0108, 1.2333) (13.4966, 0.7475) (13.4966, 0.4041) knots 0 0 0 1 2 2 2
  line L2378 (12.6674, 1.2333) -> (13.0108, 1.2333) construction
  line L2379 (13.0108, 1.2333) -> (13.4966, 0.7475) construction
  line L2380 (13.4966, 0.7475) -> (13.4966, 0.4041) construction
  line L2381 (13.4966, 0.4041) -> (13.4966, -0.8449)
  spline S697 degree 2 poles (13.4966, -0.8449) (13.4966, -1.1883) (13.0108, -1.674) (12.6674, -1.674) knots 0 0 0 1 2 2 2
  line L2382 (13.4966, -0.8449) -> (13.4966, -1.1883) construction
  line L2383 (13.4966, -1.1883) -> (13.0108, -1.674) construction
  line L2384 (13.0108, -1.674) -> (12.6674, -1.674) construction
  spline S698 degree 2 poles (2.6542, -8.9231) (2.4461, -8.9231) (2.4461, -8.715) knots 0 0 0 1 1 1
  line L2385 (2.6542, -8.9231) -> (2.4461, -8.9231) construction
  line L2386 (2.4461, -8.9231) -> (2.4461, -8.715) construction
  spline S699 degree 2 poles (2.4461, -8.715) (2.4461, -8.5068) (2.6542, -8.5068) knots 0 0 0 1 1 1
  line L2387 (2.4461, -8.715) -> (2.4461, -8.5068) construction
  line L2388 (2.4461, -8.5068) -> (2.6542, -8.5068) construction
  line L2389 (2.6542, -8.5068) -> (2.8624, -8.5068)
  spline S700 degree 2 poles (2.8624, -8.5068) (3.0567, -8.5068) (3.1712, -8.3785) knots 0 0 0 1 1 1
  line L2390 (2.8624, -8.5068) -> (3.0567, -8.5068) construction
  line L2391 (3.0567, -8.5068) -> (3.1712, -8.3785) construction
  spline S701 degree 2 poles (3.1712, -8.3785) (3.2752, -8.2605) (3.2752, -8.0905) knots 0 0 0 1 1 1
  line L2392 (3.1712, -8.3785) -> (3.2752, -8.2605) construction
  line L2393 (3.2752, -8.2605) -> (3.2752, -8.0905) construction
  spline S702 degree 2 poles (3.2752, -8.0905) (3.2752, -7.9205) (3.1712, -7.806) knots 0 0 0 1 1 1
  line L2394 (3.2752, -8.0905) -> (3.2752, -7.9205) construction
  line L2395 (3.2752, -7.9205) -> (3.1712, -7.806) construction
  spline S703 degree 2 poles (3.1712, -7.806) (3.0567, -7.6777) (2.8589, -7.6777) knots 0 0 0 1 1 1
  line L2396 (3.1712, -7.806) -> (3.0567, -7.6777) construction
  line L2397 (3.0567, -7.6777) -> (2.8589, -7.6777) construction
  line L2398 (2.8589, -7.6777) -> (2.6508, -7.6777)
  spline S704 degree 2 poles (2.6508, -7.6777) (2.3697, -7.6777) (2.1546, -7.8442) knots 0 0 0 1 1 1
  line L2399 (2.6508, -7.6777) -> (2.3697, -7.6777) construction
  line L2400 (2.3697, -7.6777) -> (2.1546, -7.8442) construction
  spline S705 degree 2 poles (2.1546, -7.8442) (2.0922, -7.8893) (2.0263, -7.8893) knots 0 0 0 1 1 1
  line L2401 (2.1546, -7.8442) -> (2.0922, -7.8893) construction
  line L2402 (2.0922, -7.8893) -> (2.0263, -7.8893) construction
  spline S706 degree 2 poles (2.0263, -7.8893) (1.943, -7.8893) (1.8181, -7.7609) (1.8181, -7.6742) knots 0 0 0 1 2 2 2
  line L2403 (2.0263, -7.8893) -> (1.943, -7.8893) construction
  line L2404 (1.943, -7.8893) -> (1.8181, -7.7609) construction
  line L2405 (1.8181, -7.7609) -> (1.8181, -7.6742) construction
  spline S707 degree 2 poles (1.8181, -7.6742) (1.8181, -7.577) (1.9048, -7.5111) knots 0 0 0 1 1 1
  line L2406 (1.8181, -7.6742) -> (1.8181, -7.577) construction
  line L2407 (1.8181, -7.577) -> (1.9048, -7.5111) construction
  spline S708 degree 2 poles (1.9048, -7.5111) (2.2275, -7.2613) (2.6508, -7.2613) knots 0 0 0 1 1 1
  line L2408 (1.9048, -7.5111) -> (2.2275, -7.2613) construction
  line L2409 (2.2275, -7.2613) -> (2.6508, -7.2613) construction
  line L2410 (2.6508, -7.2613) -> (2.8589, -7.2613)
  spline S709 degree 2 poles (2.8589, -7.2613) (3.2509, -7.2613) (3.4834, -7.5181) knots 0 0 0 1 1 1
  line L2411 (2.8589, -7.2613) -> (3.2509, -7.2613) construction
  line L2412 (3.2509, -7.2613) -> (3.4834, -7.5181) construction
  spline S710 degree 2 poles (3.4834, -7.5181) (3.6916, -7.754) (3.6916, -8.0905) knots 0 0 0 1 1 1
  line L2413 (3.4834, -7.5181) -> (3.6916, -7.754) construction
  line L2414 (3.6916, -7.754) -> (3.6916, -8.0905) construction
  spline S711 degree 2 poles (3.6916, -8.0905) (3.6916, -8.4756) (3.4314, -8.715) knots 0 0 0 1 1 1
  line L2415 (3.6916, -8.0905) -> (3.6916, -8.4756) construction
  line L2416 (3.6916, -8.4756) -> (3.4314, -8.715) construction
  spline S712 degree 2 poles (3.4314, -8.715) (3.6916, -8.9544) (3.6916, -9.3395) knots 0 0 0 1 1 1
  line L2417 (3.4314, -8.715) -> (3.6916, -8.9544) construction
  line L2418 (3.6916, -8.9544) -> (3.6916, -9.3395) construction
  spline S713 degree 2 poles (3.6916, -9.3395) (3.6916, -9.6795) (3.4834, -9.9119) knots 0 0 0 1 1 1
  line L2419 (3.6916, -9.3395) -> (3.6916, -9.6795) construction
  line L2420 (3.6916, -9.6795) -> (3.4834, -9.9119) construction
  spline S714 degree 2 poles (3.4834, -9.9119) (3.2509, -10.1686) (2.8589, -10.1686) knots 0 0 0 1 1 1
  line L2421 (3.4834, -9.9119) -> (3.2509, -10.1686) construction
  line L2422 (3.2509, -10.1686) -> (2.8589, -10.1686) construction
  line L2423 (2.8589, -10.1686) -> (2.6508, -10.1686)
  spline S715 degree 2 poles (2.6508, -10.1686) (2.2275, -10.1686) (1.9048, -9.9188) knots 0 0 0 1 1 1
  line L2424 (2.6508, -10.1686) -> (2.2275, -10.1686) construction
  line L2425 (2.2275, -10.1686) -> (1.9048, -9.9188) construction
  spline S716 degree 2 poles (1.9048, -9.9188) (1.8181, -9.8529) (1.8181, -9.7558) knots 0 0 0 1 1 1
  line L2426 (1.9048, -9.9188) -> (1.8181, -9.8529) construction
  line L2427 (1.8181, -9.8529) -> (1.8181, -9.7558) construction
  spline S717 degree 2 poles (1.8181, -9.7558) (1.8181, -9.6691) (1.943, -9.5407) (2.0263, -9.5407) knots 0 0 0 1 2 2 2
  line L2428 (1.8181, -9.7558) -> (1.8181, -9.6691) construction
  line L2429 (1.8181, -9.6691) -> (1.943, -9.5407) construction
  line L2430 (1.943, -9.5407) -> (2.0263, -9.5407) construction
  spline S718 degree 2 poles (2.0263, -9.5407) (2.0922, -9.5407) (2.1546, -9.5858) knots 0 0 0 1 1 1
  line L2431 (2.0263, -9.5407) -> (2.0922, -9.5407) construction
  line L2432 (2.0922, -9.5407) -> (2.1546, -9.5858) construction
  spline S719 degree 2 poles (2.1546, -9.5858) (2.3697, -9.7523) (2.6508, -9.7523) knots 0 0 0 1 1 1
  line L2433 (2.1546, -9.5858) -> (2.3697, -9.7523) construction
  line L2434 (2.3697, -9.7523) -> (2.6508, -9.7523) construction
  line L2435 (2.6508, -9.7523) -> (2.8589, -9.7523)
  spline S720 degree 2 poles (2.8589, -9.7523) (3.0567, -9.7523) (3.1712, -9.6205) knots 0 0 0 1 1 1
  line L2436 (2.8589, -9.7523) -> (3.0567, -9.7523) construction
  line L2437 (3.0567, -9.7523) -> (3.1712, -9.6205) construction
  spline S721 degree 2 poles (3.1712, -9.6205) (3.2752, -9.5025) (3.2752, -9.3325) knots 0 0 0 1 1 1
  line L2438 (3.1712, -9.6205) -> (3.2752, -9.5025) construction
  line L2439 (3.2752, -9.5025) -> (3.2752, -9.3325) construction
  spline S722 degree 2 poles (3.2752, -9.3325) (3.2752, -8.9613) (2.9144, -8.9231) knots 0 0 0 1 1 1
  line L2440 (3.2752, -9.3325) -> (3.2752, -8.9613) construction
  line L2441 (3.2752, -8.9613) -> (2.9144, -8.9231) construction
  line L2442 (2.9144, -8.9231) -> (2.6542, -8.9231)
  spline S723 degree 2 poles (11.5843, -9.7523) (11.7543, -9.7523) (11.9971, -9.506) (11.9971, -9.336) knots 0 0 0 1 2 2 2
  line L2443 (11.5843, -9.7523) -> (11.7543, -9.7523) construction
  line L2444 (11.7543, -9.7523) -> (11.9971, -9.506) construction
  line L2445 (11.9971, -9.506) -> (11.9971, -9.336) construction
  spline S724 degree 2 poles (11.168, -7.6777) (10.998, -7.6777) (10.7551, -7.924) (10.7551, -8.094) knots 0 0 0 1 2 2 2
  line L2446 (11.168, -7.6777) -> (10.998, -7.6777) construction
  line L2447 (10.998, -7.6777) -> (10.7551, -7.924) construction
  line L2448 (10.7551, -7.924) -> (10.7551, -8.094) construction
  line L2449 (10.7551, -8.094) -> (10.7551, -9.336)
  spline S725 degree 2 poles (10.7551, -9.336) (10.7551, -9.506) (10.998, -9.7523) (11.168, -9.7523) knots 0 0 0 1 2 2 2
  line L2450 (10.7551, -9.336) -> (10.7551, -9.506) construction
  line L2451 (10.7551, -9.506) -> (10.998, -9.7523) construction
  line L2452 (10.998, -9.7523) -> (11.168, -9.7523) construction
  line L2453 (11.168, -9.7523) -> (11.5843, -9.7523)
  line L2454 (11.5843, -10.1686) -> (11.168, -10.1686)
  spline S726 degree 2 poles (11.168, -10.1686) (10.828, -10.1686) (10.3388, -9.6829) (10.3388, -9.3395) knots 0 0 0 1 2 2 2
  line L2455 (11.168, -10.1686) -> (10.828, -10.1686) construction
  line L2456 (10.828, -10.1686) -> (10.3388, -9.6829) construction
  line L2457 (10.3388, -9.6829) -> (10.3388, -9.3395) construction
  line L2458 (10.3388, -9.3395) -> (10.3388, -8.0905)
  spline S727 degree 2 poles (10.3388, -8.0905) (10.3388, -7.747) (10.828, -7.2613) (11.168, -7.2613) knots 0 0 0 1 2 2 2
  line L2459 (10.3388, -8.0905) -> (10.3388, -7.747) construction
  line L2460 (10.3388, -7.747) -> (10.828, -7.2613) construction
  line L2461 (10.828, -7.2613) -> (11.168, -7.2613) construction
  line L2462 (11.168, -7.2613) -> (12.2053, -7.2613)
  spline S728 degree 2 poles (12.2053, -7.2613) (12.4134, -7.2613) (12.4134, -7.4695) knots 0 0 0 1 1 1
  line L2463 (12.2053, -7.2613) -> (12.4134, -7.2613) construction
  line L2464 (12.4134, -7.2613) -> (12.4134, -7.4695) construction
  line L2465 (12.4134, -7.4695) -> (12.4134, -9.3325)
  spline S729 degree 2 poles (12.4134, -9.3325) (12.4134, -9.6448) (12.7049, -9.7697) knots 0 0 0 1 1 1
  line L2466 (12.4134, -9.3325) -> (12.4134, -9.6448) construction
  line L2467 (12.4134, -9.6448) -> (12.7049, -9.7697) construction
  spline S730 degree 2 poles (12.7049, -9.7697) (12.8332, -9.8217) (12.8332, -9.9535) knots 0 0 0 1 1 1
  line L2468 (12.7049, -9.7697) -> (12.8332, -9.8217) construction
  line L2469 (12.8332, -9.8217) -> (12.8332, -9.9535) construction
  spline S731 degree 2 poles (12.8332, -9.9535) (12.8332, -10.0403) (12.7153, -10.1721) (12.6285, -10.1721) knots 0 0 0 1 2 2 2
  line L2470 (12.8332, -9.9535) -> (12.8332, -10.0403) construction
  line L2471 (12.8332, -10.0403) -> (12.7153, -10.1721) construction
  line L2472 (12.7153, -10.1721) -> (12.6285, -10.1721) construction
  spline S732 degree 2 poles (12.6285, -10.1721) (12.5834, -10.1721) (12.5383, -10.1513) knots 0 0 0 1 1 1
  line L2473 (12.6285, -10.1721) -> (12.5834, -10.1721) construction
  line L2474 (12.5834, -10.1721) -> (12.5383, -10.1513) construction
  spline S733 degree 2 poles (12.5383, -10.1513) (12.3302, -10.0611) (12.2018, -9.8946) knots 0 0 0 1 1 1
  line L2475 (12.5383, -10.1513) -> (12.3302, -10.0611) construction
  line L2476 (12.3302, -10.0611) -> (12.2018, -9.8946) construction
  spline S734 degree 2 poles (12.2018, -9.8946) (11.952, -10.1686) (11.5843, -10.1686) knots 0 0 0 1 1 1
  line L2477 (12.2018, -9.8946) -> (11.952, -10.1686) construction
  line L2478 (11.952, -10.1686) -> (11.5843, -10.1686) construction
  spline S735 degree 2 poles (15.1126, -10.1686) (14.9044, -10.1686) (14.9044, -9.9605) knots 0 0 0 1 1 1
  line L2479 (15.1126, -10.1686) -> (14.9044, -10.1686) construction
  line L2480 (14.9044, -10.1686) -> (14.9044, -9.9605) construction
  spline S736 degree 2 poles (13.6485, -10.0264) (13.6034, -10.1686) (13.4647, -10.1686) knots 0 0 0 1 1 1
  line L2481 (13.6485, -10.0264) -> (13.6034, -10.1686) construction
  line L2482 (13.6034, -10.1686) -> (13.4647, -10.1686) construction
  spline S737 degree 2 poles (13.4647, -10.1686) (13.2461, -10.1686) (13.2461, -9.9709) knots 0 0 0 1 1 1
  line L2483 (13.4647, -10.1686) -> (13.2461, -10.1686) construction
  line L2484 (13.2461, -10.1686) -> (13.2461, -9.9709) construction
  spline S738 degree 2 poles (13.2461, -9.9709) (13.2461, -9.9327) (13.26, -9.8946) knots 0 0 0 1 1 1
  line L2485 (13.2461, -9.9709) -> (13.2461, -9.9327) construction
  line L2486 (13.2461, -9.9327) -> (13.26, -9.8946) construction
  line L2487 (13.26, -9.8946) -> (14.0822, -7.4036)
  spline S739 degree 2 poles (14.0822, -7.4036) (14.1273, -7.2613) (14.2765, -7.2613) knots 0 0 0 1 1 1
  line L2488 (14.0822, -7.4036) -> (14.1273, -7.2613) construction
  line L2489 (14.1273, -7.2613) -> (14.2765, -7.2613) construction
  line L2490 (14.2765, -7.2613) -> (15.1126, -7.2613)
  spline S740 degree 2 poles (15.1126, -7.2613) (15.3207, -7.2613) (15.3207, -7.4695) knots 0 0 0 1 1 1
  line L2491 (15.1126, -7.2613) -> (15.3207, -7.2613) construction
  line L2492 (15.3207, -7.2613) -> (15.3207, -7.4695) construction
  line L2493 (15.3207, -7.4695) -> (15.3207, -9.9605)
  spline S741 degree 2 poles (15.3207, -9.9605) (15.3207, -10.1686) (15.1126, -10.1686) knots 0 0 0 1 1 1
  line L2494 (15.3207, -9.9605) -> (15.3207, -10.1686) construction
  line L2495 (15.3207, -10.1686) -> (15.1126, -10.1686) construction
  spline S742 degree 2 poles (-17.4874, -21.78) (-17.3174, -21.78) (-17.0746, -21.5337) (-17.0746, -21.3637) knots 0 0 0 1 2 2 2
  line L2496 (-17.4874, -21.78) -> (-17.3174, -21.78) construction
  line L2497 (-17.3174, -21.78) -> (-17.0746, -21.5337) construction
  line L2498 (-17.0746, -21.5337) -> (-17.0746, -21.3637) construction
  spline S743 degree 2 poles (-17.9037, -19.7053) (-18.0737, -19.7053) (-18.3166, -19.9517) (-18.3166, -20.1217) knots 0 0 0 1 2 2 2
  line L2499 (-17.9037, -19.7053) -> (-18.0737, -19.7053) construction
  line L2500 (-18.0737, -19.7053) -> (-18.3166, -19.9517) construction
  line L2501 (-18.3166, -19.9517) -> (-18.3166, -20.1217) construction
  line L2502 (-18.3166, -20.1217) -> (-18.3166, -21.3637)
  spline S744 degree 2 poles (-18.3166, -21.3637) (-18.3166, -21.5337) (-18.0737, -21.78) (-17.9037, -21.78) knots 0 0 0 1 2 2 2
  line L2503 (-18.3166, -21.3637) -> (-18.3166, -21.5337) construction
  line L2504 (-18.3166, -21.5337) -> (-18.0737, -21.78) construction
  line L2505 (-18.0737, -21.78) -> (-17.9037, -21.78) construction
  line L2506 (-17.9037, -21.78) -> (-17.4874, -21.78)
  line L2507 (-17.4874, -22.1963) -> (-17.9037, -22.1963)
  spline S745 degree 2 poles (-17.9037, -22.1963) (-18.2437, -22.1963) (-18.7329, -21.7106) (-18.7329, -21.3672) knots 0 0 0 1 2 2 2
  line L2508 (-17.9037, -22.1963) -> (-18.2437, -22.1963) construction
  line L2509 (-18.2437, -22.1963) -> (-18.7329, -21.7106) construction
  line L2510 (-18.7329, -21.7106) -> (-18.7329, -21.3672) construction
  line L2511 (-18.7329, -21.3672) -> (-18.7329, -20.1182)